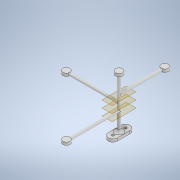
# Autodesk Inventor part: VICON_HOLDER
Saved by Autodesk Inventor 2022 (Build 260153000, 153)
## iProperties
Created: 2023-03-29
Part Number: VICON_HOLDER
Material: Generic
Document SubType Name: Modeling
Designer: ARRF
Density: 1 g/cm^3
Appearance: Default
Author: ARRF
Autodesk Inventor part; units mm, degrees
ref_plane "YZ Plane" through (0, 0, 0) normal (1, 0, 0) x (0, 1, 0)
ref_plane "XZ Plane" through (0, 0, 0) normal (0, 1, 0) x (-1, 0, 0)
ref_plane "XY Plane" through (0, 0, 0) normal (0, 0, 1) x (1, 0, 0)
sketch "Sketch1" plane through (0, 0, 0) normal (0, 1, 0) x (-1, 0, 0)
  circle A0 centre (0, 0) radius 14
  circle A1 centre (0, 9) radius 1.75
  circle A2 centre (0, -9) radius 1.75
  line L0 (0, 9) -> (0, -9) construction
  line L1 (-6.5, 9) -> (-6.5, -9)
  line L2 (6.5, -9) -> (6.5, 9)
  arc A3 (6.5, 9) -> (-6.5, 9) centre (0, 9) ccw
  arc A4 (-6.5, -9) -> (6.5, -9) centre (0, -9) ccw
  point P0 (0, 0)
  dimension "d0" = 28
  dimension "d1" = 3.5
  dimension "d2" = 3.5
  dimension "d3" = 18
  dimension "d4" = 9
  dimension "d5" = 13
  constraints: 8 end point, 5 centre point, 4 point on circle, 4 tangent, 1 coincident, 1 midpoint, 1 parallel, 1 vertical
  measures "d0" diameter of A0
  measures "d1" diameter of A1
  measures "d2" diameter of A2
  measures "d3" distance of L0.end L0.start
  measures "d4" distance of point (0, 0) L0.start
  measures "d5" diameter of A4
extrude "Extrusion1" add sketch "Sketch1" along normal blind 4 contours A3 L2 A4 A0 L1 | A0 A3 | A4 A0
sketch "Sketch2" plane through (0, 4, 0) normal (0, 1, 0) x (1, 0, 0)
  circle A0 centre (0, 0) radius 2
  dimension "d8" = 4
  constraints: 1 centre point, 1 coincident
  measures "d8" diameter of A0
extrude "Extrusion2" add sketch "Sketch2" along normal blind 75
sketch "Sketch3" plane through (0, 0, 0) normal (0, 0, 1) x (1, 0, 0)
  line L0 (0, 0) -> (-51.423, 61.2836)
  line L1 (0, 0) -> (80, 0) construction
  dimension "d11" = 80
  dimension "d12" = 130
  constraints: 4 end point, 1 equal length, 1 horizontal
  measures "d11" distance of L0.start L0.end
  measures "d12" angle of L1 L0
sketch "Sketch4" plane through (0, 0, 0) normal (1, 0, 0) x (0, 1, 0)
  line L0 (0, 0) -> (40, 69.282)
  line L1 (0, 0) -> (80, 0) construction
  dimension "d13" = 80
  dimension "d14" = 60
  constraints: 4 end point, 1 equal length, 1 horizontal
  measures "d13" distance of L0.start L0.end
  measures "d14" angle of L1 L0
sketch "Sketch5" plane through (0, 0, 0) normal (1, 0, 0) x (0, 1, 0)
  line L0 (50, 0.1781) -> (75, -43.1232)
  line L1 (50, 0.1781) -> (100, 0.1781) construction
  line L2 (0, 9) -> (0, -9) projected
  point P0 (0, 0)
  dimension "d15" = 50
  dimension "d16" = 60
  dimension "d17" = 50
  constraints: 4 end point, 1 equal length, 1 horizontal
  measures "d15" distance of L0.start L0.end
  measures "d16" angle of L0 L1
  measures "d17" distance from line of L2 L0.start
sketch "Sketch9" plane through (0, 0, 0) normal (0, 0, 1) x (1, 0, 0)
  circle A0 centre (0, 30) radius 2
  line L0 (6.5, 0) -> (-6.5, 0) projected
  point P0 (0, 0)
  dimension "d25" = 4
  dimension "d26" = 30
  constraints: 1 centre point
  measures "d25" diameter of A0
  measures "d26" distance from line of L0 A0.centre
extrude "Extrusion3" add sketch "Sketch9" along normal blind 75
sketch "Sketch10" plane through (0, 0, 0) normal (0, 0, 1) x (1, 0, 0)
  circle A0 centre (0, 50) radius 2
  point P0 (0, 0)
  dimension "d29" = 4
  dimension "d30" = 50
  constraints: 1 centre point
  measures "d29" diameter of A0
  measures "d30" distance of point (0, 0) A0.centre
extrude "Extrusion4" add sketch "Sketch10" against normal blind 65
sketch "Sketch11" plane through (0, 0, 0) normal (1, 0, 0) x (0, 1, 0)
  circle A0 centre (40, 0) radius 2
  point P0 (0, 0)
  dimension "d33" = 4
  dimension "d36" = 40
  constraints: 1 centre point
  measures "d33" diameter of A0
  measures "d36" distance of point (0, 0) A0.centre
extrude "Extrusion5" add sketch "Sketch11" against normal blind 75
ref_plane "Work Plane2" through (0, 28, 0) normal (0, 1, 0) x (1, 0, 0)
sketch "Sketch12" plane through (0, 28, 0) normal (0, 1, 0) x (1, 0, 0)
  line L0 (-2, -75) -> (2, -75) projected
  circle A0 centre (0, -75) radius 5
  point P0 (0, 0)
  dimension "d38" = 10
  constraints: 1 centre point, 1 midpoint
  measures "d38" diameter of A0
extrude "Extrusion6" add sketch "Sketch12" along normal blind 4
ref_plane "Work Plane3" through (0, 38, 0) normal (0, 1, 0) x (1, 0, 0)
sketch "Sketch13" plane through (0, 38, 0) normal (0, 1, 0) x (1, 0, 0)
  line L0 (-75, 2) -> (-75, -2) projected
  circle A0 centre (-75, 0) radius 5
  point P0 (0, 0)
  dimension "d42" = 10
  constraints: 1 centre point, 1 midpoint
  measures "d42" diameter of A0
extrude "Extrusion7" add sketch "Sketch13" along normal blind 4
ref_plane "Work Plane4" through (0, 48, 0) normal (0, 1, 0) x (1, 0, 0)
sketch "Sketch14" plane through (0, 48, 0) normal (0, 1, 0) x (1, 0, 0)
  line L0 (2, 65) -> (-2, 65) projected
  circle A0 centre (0, 65) radius 5
  point P0 (0, 0)
  dimension "d46" = 10
  constraints: 1 centre point, 1 midpoint
  measures "d46" diameter of A0
extrude "Extrusion8" add sketch "Sketch14" along normal blind 4
sketch "Sketch15" plane through (0, 79, 0) normal (0, 1, 0) x (1, 0, 0)
  arc A0 (2, 0) -> (-2, 0) centre (0, 0) ccw projected
  circle A1 centre (0, 0) radius 5
  dimension "d49" = 10
  constraints: 1 centre point, 1 coincident
  measures "d49" diameter of A1
extrude "Extrusion9" add sketch "Sketch15" against normal blind 4
fillet "Fillet1" radius 4 1 edges at (-2, 4, 0)
sketch "Sketch6" plane through (0, 4, 0) normal (0, 1, 0) x (1, 0, 0)
  circle A0 centre (0, 0) radius 2 projected
sketch "Sketch7" plane through (0, 4, 0) normal (0, 1, 0) x (1, 0, 0)
  circle A0 centre (0, 0) radius 2 projected
sketch "Sketch8" plane through (0, 50, 0) normal (0, 1, 0) x (1, 0, 0)
  circle A0 centre (0, 0) radius 2 projected
body "Solid1"
